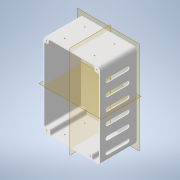
# Autodesk Inventor part: Omniscope_sidewalls_v0
Saved by Autodesk Inventor 2022 (Build 260153000, 153)
## iProperties
Created: 2022-05-25
Part Number: Omniscope_sidewalls_v0
Material: Generisch
Document SubType Name: Modeling
Designer: diederichbenedict
Density: 1 g/cm^3
Appearance: Vorgabe
Author: diederichbenedict
Autodesk Inventor part; units mm, degrees
ref_plane "YZ Plane" through (0, 0, 0) normal (1, 0, 0) x (0, 1, 0)
ref_plane "XZ Plane" through (0, 0, 0) normal (0, 1, 0) x (-1, 0, 0)
ref_plane "XY Plane" through (0, 0, 0) normal (0, 0, 1) x (1, 0, 0)
ref_plane "Arbeitsebene1" through (0, 0, 0) normal (0, 0, 1) x (1, 0, 0)
sketch "Skizze1" plane through (0, 0, 0) normal (0, 0, 1) x (1, 0, 0)
  circle A0 centre (37.75, -58.75) radius 1.4 projected
  circle A1 centre (37.75, 58.75) radius 1.4 projected
  circle A2 centre (-37.75, 58.75) radius 1.4 projected
  circle A3 centre (-37.75, -58.75) radius 1.4 projected
  circle A4 centre (-28.35, -47.25) radius 8 projected
  circle A5 centre (-28.35, -28.35) radius 8 projected
  circle A6 centre (-28.35, -9.45) radius 8 projected
  circle A7 centre (-28.35, 9.45) radius 8 projected
  circle A8 centre (-28.35, 28.35) radius 8 projected
  circle A9 centre (-28.35, 47.25) radius 8 projected
  circle A10 centre (-9.45, -47.25) radius 8 projected
  circle A11 centre (-9.45, -28.35) radius 8 projected
  circle A12 centre (-9.45, -9.45) radius 8 projected
  circle A13 centre (-9.45, 9.45) radius 8 projected
  circle A14 centre (-9.45, 28.35) radius 8 projected
  circle A15 centre (-9.45, 47.25) radius 8 projected
  circle A16 centre (9.45, -47.25) radius 8 projected
  circle A17 centre (9.45, -28.35) radius 8 projected
  circle A18 centre (9.45, -9.45) radius 8 projected
  circle A19 centre (9.45, 9.45) radius 8 projected
  circle A20 centre (9.45, 28.35) radius 8 projected
  circle A21 centre (9.45, 47.25) radius 8 projected
  circle A22 centre (28.35, -47.25) radius 8 projected
  circle A23 centre (28.35, -28.35) radius 8 projected
  circle A24 centre (28.35, -9.45) radius 8 projected
  circle A25 centre (28.35, 9.45) radius 8 projected
  circle A26 centre (28.35, 28.35) radius 8 projected
  arc A27 (37.75, -63.75) -> (42.75, -58.75) centre (37.75, -58.75) ccw projected
  line L0 (42.75, -58.75) -> (42.75, 58.75) projected
  arc A28 (42.75, 58.75) -> (37.75, 63.75) centre (37.75, 58.75) ccw projected
  line L1 (37.75, 63.75) -> (-37.75, 63.75) projected
  arc A29 (-37.75, 63.75) -> (-42.75, 58.75) centre (-37.75, 58.75) ccw projected
  line L2 (-42.75, 58.75) -> (-42.75, -58.75) projected
  arc A30 (-42.75, -58.75) -> (-37.75, -63.75) centre (-37.75, -58.75) ccw projected
  line L3 (-37.75, -63.75) -> (37.75, -63.75) projected
  circle A31 centre (28.35, 47.25) radius 8 projected
  line L4 (41.25, 58.75) -> (41.25, -58.75)
  arc A32 (37.75, -62.25) -> (41.25, -58.75) centre (37.75, -58.75) ccw
  line L5 (37.75, -62.25) -> (-37.75, -62.25)
  arc A33 (-41.25, -58.75) -> (-37.75, -62.25) centre (-37.75, -58.75) ccw
  line L6 (-41.25, -58.75) -> (-41.25, 58.75)
  arc A34 (-37.75, 62.25) -> (-41.25, 58.75) centre (-37.75, 58.75) ccw
  line L7 (-37.75, 62.25) -> (37.75, 62.25)
  arc A35 (41.25, 58.75) -> (37.75, 62.25) centre (37.75, 58.75) ccw
  line L8 (-34.75, 62.25) -> (-34.75, 55.75)
  line L9 (-34.75, 55.75) -> (-41.25, 55.75)
  line L10 (-32.5541, -62.25) -> (-32.5541, -54.8048)
  line L11 (-32.5541, -54.8048) -> (-41.25, -54.8048)
  line L12 (41.25, 55.25) -> (34.25, 55.25)
  line L13 (34.25, 55.25) -> (34.25, 62.25)
  line L14 (31.25, -62.25) -> (24.25, -62.25)
  line L15 (24.25, -62.25) -> (24.25, -55.25)
  line L16 (24.25, -55.25) -> (31.25, -55.25)
  line L17 (31.25, -55.25) -> (31.25, -62.25)
  circle A36 centre (28.25, -59.25) radius 1.4
  point P0 (0, 0)
  point P1 (24.25, -62.25)
  dimension "d0" = 1.5
  dimension "d1" = 3
  dimension "d2" = 3
  dimension "d5" = 7
  dimension "d6" = 7
  dimension "d7" = 7
  dimension "d8" = 7
  dimension "d9" = 10
  dimension "d10" = 2.8
  constraints: 28 end point, 8 point on circle, 7 point on line, 5 centre point, 4 perpendicular, 2 horizontal, 2 parallel, 2 vertical, 7 other
  measures "d0" distance between parallel lines of L0 L4
  measures "d1" distance from line of A2.centre L8
  measures "d2" distance from line of A2.centre L9
  measures "d5" distance between parallel lines of L13 L4
  measures "d6" distance between parallel lines of L7 L12
  measures "d7" distance of L15.end L16.end
  measures "d8" distance of L14.end L15.end
  measures "d9" distance between parallel lines of L17 L4
  measures "d10" diameter of A36
ref_plane "Arbeitsebene2" through (23.1342, 37.0359, 54) normal (0, 0, 1) x (0.819152, 0.5735764, 0)
extrude "Extrusion1" add sketch "Skizze1" along normal blind 55 contours L16 L17 L5 L15 | L5 A33 L6 L11 L10 | L12 L13 L7 A35 L4 | L6 A34 L7 L8 L9 | L3 A30 L2 A29 L1 A28 L0 A27
fillet "Rundung1" radius 2 13 edges at (-32.5541, -54.8048, 27.5) (-41.25, -54.8048, 27.5) (-32.5541, -62.25, 27.5) (24.25, -62.25, 27.5) (24.25, -55.25, 27.5) (31.25, -55.25, 27.5) (31.25, -62.25, 27.5) (41.25, 55.25, 27.5) (34.25, 55.25, 27.5) (34.25, 62.25, 27.5) (-34.75, 55.75, 27.5) (-41.25, 55.75, 27.5) (-34.75, 62.25, 27.5)
sketch "Skizze4" plane through (42.75, -58.75, 0) normal (1, 0, 0) x (0, 0, -1)
  line L0 (-43.7633, 6.3718) -> (-13.7057, 6.3718) construction
  line L1 (0, 5.9452) -> (-55, 5.9452) projected
  line L2 (-43.7633, 3.3718) -> (-13.7057, 3.3718)
  line L3 (-13.7057, 9.3718) -> (-43.7633, 9.3718)
  arc A0 (-43.7633, 9.3718) -> (-43.7633, 3.3718) centre (-43.7633, 6.3718) ccw
  arc A1 (-13.7057, 3.3718) -> (-13.7057, 9.3718) centre (-13.7057, 6.3718) ccw
  point P0 (0, 58.75)
  point P1 (-36.8275, 7.2035)
  point P2 (-36.1925, 26.1035)
  point P3 (-36.1925, 45.0035)
  point P4 (-36.1925, 63.9035)
  point P5 (-36.1925, 82.8035)
  point P6 (-36.1925, 101.7035)
  point P7 (-28.7345, 6.3718)
  dimension "d29" = 6
  constraints: 8 end point, 4 point on circle, 4 tangent, 2 centre point, 2 parallel, 1 midpoint, 6 other
  measures "d29" distance between parallel lines of L3 L2
extrude "Extrusion4" cut sketch "Skizze4" against normal blind 55
pattern_linear "Rechteckige Anordnung2" count 6 spacing 18.9 along (0, 1, 0) of "Extrusion4"
ref_plane "Arbeitsebene3" through (0, -58.75, 0) normal (1, 0, 0) x (0, 0, -1)
ref_plane "Arbeitsebene4" through (-37.75, 0, 0) normal (0, 1, 0) x (1, 0, 0)
sketch "Skizze5" plane through (-37.75, 63.75, 0) normal (0, 1, 0) x (1, 0, 0)
  line L0 (75.5, 0) -> (0, 0) projected
  line L1 (0, 0) -> (0, -55) projected
  line L2 (75.5, -55) -> (0, -55) projected
  line L3 (75.5, 0) -> (75.5, -55) projected
  line L4 (60.25, -42.5) -> (15.25, -42.5)
  line L5 (15.25, -42.5) -> (15.25, -12.5)
  line L6 (15.25, -12.5) -> (60.25, -12.5)
  line L7 (60.25, -12.5) -> (60.25, -42.5)
  line L8 (60.25, -42.5) -> (15.25, -12.5) construction
  line L9 (15.25, -42.5) -> (60.25, -12.5) construction
  point P0 (37.75, 0)
  point P1 (52.5946, -34.1859)
  point P2 (37.75, -27.5)
  dimension "d35" = 45
  dimension "d36" = 30
  constraints: 12 end point, 2 midpoint, 2 parallel, 1 horizontal, 1 perpendicular, 1 other
  measures "d35" distance of L5.end L6.end
  measures "d36" distance of L4.end L5.end
hole "Bohrung1" at (22.5, 63.75, 42.5) at (-22.5, 63.75, 42.5) at (-22.5, 63.75, 12.5) at (22.5, 63.75, 12.5) direction (0, -1, 0) diameter 2.8 end through all
